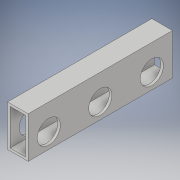
# Autodesk Inventor part: Clamp Arms
Saved by Autodesk Inventor 2018 (Build 220112000, 112)
## iProperties
Created: 2018-02-03
Part Number: Clamp Arms
Material: Generic
Document SubType Name: Modeling
Designer: Luke
Density: 1 g/cm^3
Appearance: Default
Author: Luke
Autodesk Inventor part; units mm, degrees
ref_plane "YZ Plane" through (0, 0, 0) normal (1, 0, 0) x (0, 1, 0)
ref_plane "XZ Plane" through (0, 0, 0) normal (0, 1, 0) x (-1, 0, 0)
ref_plane "XY Plane" through (0, 0, 0) normal (0, 0, 1) x (1, 0, 0)
sketch "Sketch1" plane through (0, 0, 0) normal (0, 0, 1) x (1, 0, 0)
  line L0 (0, 0) -> (-25.4, 0)
  line L1 (-25.4, 0) -> (-25.4, 50.8)
  line L2 (-25.4, 50.8) -> (0, 50.8)
  line L3 (0, 50.8) -> (0, 0)
  line L4 (-22.225, 3.175) -> (-3.175, 3.175)
  line L5 (-3.175, 3.175) -> (-3.175, 47.625)
  line L6 (-3.175, 47.625) -> (-22.225, 47.625)
  line L7 (-22.225, 47.625) -> (-22.225, 3.175)
  dimension "d0" = 25.4
  dimension "d1" = 50.8
  dimension "d2" = 3.175
  constraints: 16 end point, 4 parallel, 2 perpendicular, 1 horizontal, 3 other
  measures "d0" distance of L1.end L2.end
  measures "d1" distance of L0.end L1.end
  measures "d2" distance between parallel lines of L0 L4
extrude "Extrusion1" add sketch "Sketch1" along normal blind 177.8
sketch "Sketch2" plane through (0, 0, 0) normal (1, 0, 0) x (0, 0, -1)
  circle A0 centre (-152.4, 19.05) radius 14.2875
  circle A1 centre (-25.4, 19.05) radius 14.2875
  circle A2 centre (-88.9, 19.05) radius 14.2875
  line L0 (-177.8, 0) -> (-177.8, 50.8) projected
  line L1 (0, 50.8) -> (0, 0) projected
  line L2 (0, 50.8) -> (-177.8, 50.8) projected
  line L3 (0, 0) -> (-177.8, 0) projected
  dimension "d5" = 28.575
  dimension "d6" = 28.575
  dimension "d7" = 28.575
  dimension "d8" = 25.4
  dimension "d9" = 25.4
  dimension "d10" = 31.75
  dimension "d11" = 31.75
  dimension "d12" = 19.05
  dimension "a" = 63.5
  dimension "d14" = 63.5
  constraints: 3 centre point
  measures "d5" diameter of A1
  measures "d6" diameter of A2
  measures "d7" diameter of A0
  measures "d8" distance from line of L0 A0.centre
  measures "d9" distance from line of L1 A1.centre
  measures "d10" distance from line of L2 A1.centre
  measures "d11" distance from line of L2 A0.centre
  measures "d12" distance from line of L3 A2.centre
  measures "a" distance of A0.centre A2.centre
  measures "d14" distance of A2.centre A1.centre
extrude "Extrusion2" cut sketch "Sketch2" against normal blind 209.3722 contours A0 | A1 | A2
body "Solid1"
